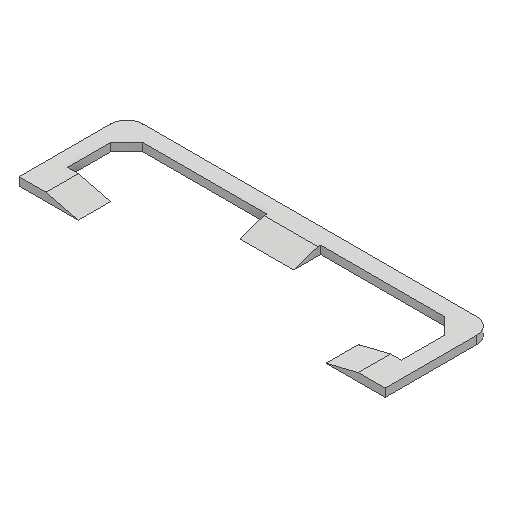
# Autodesk Inventor part: 3DP_PLA_Back_slider
Saved by Autodesk Inventor 2025 (Build 290162010, 162A)
## iProperties
Created: 2016-05-02
Part Number: 3DP_PLA_Back_slider
Material: Ogólny
Document SubType Name: Modeling
Designer: Andrzej
Density: 1 g/cm^3
Appearance: Domyślna
Mass: 0.597956 g
Surface Area: 12.3004 cm^2
Volume: 0.597956 cm^3
Author: Andrzej
Autodesk Inventor part; units mm, degrees
ref_plane "YZ Plane" through (0, 0, 0) normal (1, 0, 0) x (0, 1, 0)
ref_plane "XZ Plane" through (0, 0, 0) normal (0, 1, 0) x (-1, 0, 0)
ref_plane "XY Plane" through (0, 0, 0) normal (0, 0, 1) x (1, 0, 0)
sketch "Szkic1" plane through (0, 0, 0) normal (0, 0, 1) x (1, 0, 0)
  line L0 (-20.164, -13.0508) -> (-20.164, 6.9492)
  line L1 (-20.164, 6.9492) -> (47.836, 6.9492)
  line L2 (47.836, 6.9492) -> (47.836, -13.0508)
  line L3 (-20.164, -13.0508) -> (-17.164, -13.0508)
  line L4 (-17.164, -13.0508) -> (-17.164, 3.9492)
  line L5 (-17.164, 3.9492) -> (44.836, 3.9492)
  line L6 (44.836, 3.9492) -> (44.836, -13.0508)
  line L7 (44.836, -13.0508) -> (47.836, -13.0508)
  line L8 (8.836, 3.9492) -> (8.836, -1.0508)
  line L9 (18.836, 3.9492) -> (18.836, -1.0508)
  line L10 (-9.164, -13.0508) -> (-9.164, -7.0508)
  line L11 (36.836, -13.0508) -> (36.836, -7.0508)
  line L12 (8.836, -1.0508) -> (18.836, -1.0508)
  line L13 (44.836, -7.0508) -> (36.836, -7.0508)
  line L14 (-9.164, -7.0508) -> (-17.164, -7.0508)
  line L15 (-17.164, -13.0508) -> (-9.164, -13.0508)
  line L16 (36.836, -13.0508) -> (44.836, -13.0508)
  point P0 (0, 0)
  dimension "d0" = 20
  dimension "d1" = 68
  dimension "d2" = 20
  dimension "d3" = 3
  dimension "d4" = 3
  dimension "d5" = 3
  dimension "d7" = 10
  dimension "d8" = 62
  dimension "d9" = 26
  dimension "d10" = 8
  dimension "d11" = 8
  dimension "d12" = 5
  constraints: 34 end point, 16 perpendicular, 5 point on line, 3 horizontal, 1 vertical
  measures "d0" distance of L0.start L0.end
  measures "d1" distance of L0.end L1.end
  measures "d2" distance of L1.end L2.end
  measures "d3" distance of L0.start L3.end
  measures "d4" distance between parallel lines of L1 L5
  measures "d5" distance between parallel lines of L2 L6
  measures "d7" distance between parallel lines of L9 L8
  measures "d8" distance between parallel lines of L6 L4
  measures "d9" distance between parallel lines of L4 L8
  measures "d10" distance between parallel lines of L4 L10
  measures "d11" distance between parallel lines of L6 L11
  measures "d12" distance between parallel lines of L5 L12
extrude "Wyciągnięcie proste1" add sketch "Szkic1" along normal blind 1.5 contours L0 L1 L2 L7 L6 L5 L4 L3
extrude "Wyciągnięcie proste2" add sketch "Szkic1" along normal blind 1.5 contours L4 L14 L10 L15 | L16 L11 L13 L6 | L5 L9 L12 L8
chamfer "Faza1" distance 4.5 distance2 1.5 1 edges at (13.836, -1.0508, 1.5) measured on face at (13.836, -0.5508, 1.5)
chamfer "Faza2" distance 6 distance2 1.5 1 edges at (-9.164, -10.0508, 1.5) measured on face at (-9.664, -10.0508, 1.5)
chamfer "Faza3" distance 6 distance2 1.5 1 edges at (36.836, -10.0508, 1.5) measured on face at (37.336, -10.0508, 1.5)
fillet "Zaokrąglenie2" radius 3 2 edges at (-20.164, 6.9492, 0.75) (47.836, 6.9492, 0.75)
chamfer "Faza4" distance 3 angle 45 2 edges at (-17.164, 3.9492, 0.75) (44.836, 3.9492, 0.75)
equation "\"d2\" = d0"
equation "\"d4\" = d3"
equation "\"d5\" = d3"
equation "\"d9\" = -0.5 * d7 + 0.5 * d8"
